1f435360-b7cd-40b3-95bb-e526e7d264a0 (Autodesk Fusion 360 design; units mm, degrees)
Autodesk Fusion 360 part; units mm, degrees
sketch "Sketch1" plane through (0, 0, 0) normal (0, 0, 1) x (1, 0, 0)
  circle A0 centre (0, 0) radius 6.35
  circle A1 centre (0, 0) radius 7.9375
  dimension "d1" = 12.7
  dimension "d2" = 15.875
  measures "d1" diameter of A0
  measures "d2" diameter of A1
extrude "Extrude1" add sketch "Sketch1" along normal blind 25.4
sketch "Sketch2" plane through (0, 0, 0) normal (0, 0, -1) x (-1, 0, 0)
  circle A0 centre (0, 0) radius 7.9375
  circle A1 centre (0, 0) radius 11.1125
  circle A2 centre (0, 0) radius 6.35
  dimension "d5" = 22.225
  measures "d5" diameter of A1
extrude "Extrude2" add sketch "Sketch2" against normal blind 3.175 contours A1
equation "d1 = Shaft_ID"
equation "d2 = Housing_ID"
equation "d3 = Length"
equation "d5 = Flange_OD"
equation "d6 = FlangeT"
equation "Shaft_ID = ( 1 / 2 ) * 1 in"
equation "Housing_ID = ( 5 / 8 ) * 1 in"
equation "FlangeT = ( -1 / 8 ) * 1 in"
equation "Length = 1 in"
equation "Flange_OD = ( 7 / 8 ) * 1 in"
